Autodesk Inventor part; units mm, degrees
(part 2 of 3)
  spline S242 degree 2 poles (12.9177, 0.2255) (13.1098, 0.3179) (13.6422, 0.3908) (13.9485, 0.4102) knots 0 0 0 1 2 2 2
  line L379 (13.9485, 0.4102) -> (13.9485, 0.4224)
  spline S243 degree 2 poles (13.9485, 0.4224) (13.9485, 0.6096) (13.6714, 0.753) (13.3942, 0.753) knots 0 0 0 1 2 2 2
  spline S244 degree 2 poles (13.3942, 0.753) (13.2702, 0.753) (12.9347, 0.6631) (12.7767, 0.5926) knots 0 0 0 1 2 2 2
  line L380 (12.7767, 0.5926) -> (12.7159, 0.5926)
  line L381 (12.7159, 0.5926) -> (12.7159, 1.1396)
  spline S245 degree 2 poles (12.7159, 1.1396) (12.8205, 1.1688) (13.2872, 1.2514) (13.5255, 1.2514) knots 0 0 0 1 2 2 2
  spline S246 degree 2 poles (13.5255, 1.2514) (14.109, 1.2514) (14.6438, 0.8624) (14.6438, 0.4637) knots 0 0 0 1 2 2 2
  line L382 (14.6438, 0.4637) -> (14.6438, -1.0752)
  line L383 (14.6438, -1.0752) -> (13.9436, -1.0752)
  line L384 (13.9436, -1.0752) -> (13.9436, -0.8345)
  line L385 (13.9436, -0.4844) -> (13.9436, -0.0152)
  spline S247 degree 2 poles (13.9436, -0.0152) (13.7637, -0.0322) (13.5425, -0.059) (13.4355, -0.0979) knots 0 0 0 1 2 2 2
  spline S248 degree 2 poles (13.4355, -0.0979) (13.3407, -0.1295) (13.2386, -0.2607) (13.2386, -0.3677) knots 0 0 0 1 2 2 2
  spline S249 degree 2 poles (13.2386, -0.3677) (13.2386, -0.5257) (13.4112, -0.6449) (13.579, -0.6449) knots 0 0 0 1 2 2 2
  spline S250 degree 2 poles (13.579, -0.6449) (13.6714, -0.6449) (13.8658, -0.5598) (13.9436, -0.4844) knots 0 0 0 1 2 2 2
  line L386 (17.4323, -1.0752) -> (16.5936, -1.0752)
  line L387 (16.5936, -1.0752) -> (15.9809, -0.093)
  line L388 (15.9809, -0.093) -> (15.8715, -0.2389)
  line L389 (15.8715, -0.2389) -> (15.8715, -1.0752)
  line L390 (15.8715, -1.0752) -> (15.1665, -1.0752)
  line L391 (15.1665, -1.0752) -> (15.1665, 2.0585)
  line L392 (15.1665, 2.0585) -> (15.8715, 2.0585)
  line L393 (15.8715, 2.0585) -> (15.8715, 0.3033)
  line L394 (15.8715, 0.3033) -> (16.5401, 1.1882)
  line L395 (16.5401, 1.1882) -> (17.3739, 1.1882)
  line L396 (17.3739, 1.1882) -> (16.5814, 0.2133)
  line L397 (16.5814, 0.2133) -> (17.4323, -1.0752)
  spline S251 degree 2 poles (-23.8578, -3.9603) (-23.8578, -4.1694) (-23.9915, -4.5486) (-24.1155, -4.675) knots 0 0 0 1 2 2 2
  spline S252 degree 2 poles (-24.1155, -4.675) (-24.1909, -4.7553) (-24.3757, -4.8865) (-24.4851, -4.9327) knots 0 0 0 1 2 2 2
  spline S253 degree 2 poles (-24.4851, -4.9327) (-24.5969, -4.9789) (-24.857, -5.0324) (-25.0175, -5.0324) knots 0 0 0 1 2 2 2
  line L398 (-25.0175, -5.0324) -> (-25.4113, -5.0324)
  line L399 (-25.4113, -5.0324) -> (-25.4113, -6.0146)
  line L400 (-25.4113, -6.0146) -> (-26.165, -6.0146)
  line L401 (-26.165, -6.0146) -> (-26.165, -3.0146)
  line L402 (-26.165, -3.0146) -> (-25.0004, -3.0146)
  spline S254 degree 2 poles (-25.0004, -3.0146) (-24.7427, -3.0146) (-24.3659, -3.1094) (-24.2128, -3.2115) knots 0 0 0 1 2 2 2
  spline S255 degree 2 poles (-24.2128, -3.2115) (-24.0426, -3.3258) (-23.8578, -3.7002) (-23.8578, -3.9603) knots 0 0 0 1 2 2 2
  spline S256 degree 2 poles (-24.6309, -3.9797) (-24.6309, -3.8509) (-24.7525, -3.6686) (-24.8351, -3.6345) knots 0 0 0 1 2 2 2
  spline S257 degree 2 poles (-24.8351, -3.6345) (-24.9421, -3.5883) (-25.1366, -3.5737) (-25.3043, -3.5737) knots 0 0 0 1 2 2 2
  line L403 (-25.3043, -3.5737) -> (-25.4113, -3.5737)
  line L404 (-25.4113, -3.5737) -> (-25.4113, -4.4733)
  line L405 (-25.4113, -4.4733) -> (-25.3578, -4.4733)
  spline S258 degree 2 poles (-25.3578, -4.4733) (-25.2533, -4.4733) (-25.0637, -4.4684) (-24.9932, -4.4562) knots 0 0 0 1 2 2 2
  spline S259 degree 2 poles (-24.9932, -4.4562) (-24.9324, -4.4465) (-24.7987, -4.3882) (-24.7622, -4.3517) knots 0 0 0 1 2 2 2
  spline S260 degree 2 poles (-24.7622, -4.3517) (-24.6844, -4.2788) (-24.6309, -4.1159) (-24.6309, -3.9797) knots 0 0 0 1 2 2 2
  spline S261 degree 2 poles (-21.3246, -4.8841) (-21.3246, -5.4433) (-21.9348, -6.0851) (-22.4915, -6.0851) knots 0 0 0 1 2 2 2
  spline S262 degree 2 poles (-22.4915, -6.0851) (-23.0458, -6.0851) (-23.6609, -5.4433) (-23.6609, -4.8841) knots 0 0 0 1 2 2 2
  spline S263 degree 2 poles (-23.6609, -4.8841) (-23.6609, -4.3201) (-23.0458, -3.6807) (-22.4915, -3.6807) knots 0 0 0 1 2 2 2
  spline S264 degree 2 poles (-22.4915, -3.6807) (-21.9372, -3.6807) (-21.3246, -4.3225) (-21.3246, -4.8841) knots 0 0 0 1 2 2 2
  spline S265 degree 2 poles (-22.0466, -4.889) (-22.0466, -4.6872) (-22.1123, -4.4173) (-22.1706, -4.3371) knots 0 0 0 1 2 2 2
  spline S266 degree 2 poles (-22.1706, -4.3371) (-22.2338, -4.252) (-22.3919, -4.1864) (-22.4915, -4.1864) knots 0 0 0 1 2 2 2
  spline S267 degree 2 poles (-22.4915, -4.1864) (-22.5888, -4.1864) (-22.7419, -4.2447) (-22.8051, -4.3274) knots 0 0 0 1 2 2 2
  spline S268 degree 2 poles (-22.8051, -4.3274) (-22.8659, -4.4052) (-22.9389, -4.6799) (-22.9389, -4.889) knots 0 0 0 1 2 2 2
  spline S269 degree 2 poles (-22.9389, -4.889) (-22.9389, -5.0956) (-22.8708, -5.3509) (-22.8149, -5.4287) knots 0 0 0 1 2 2 2
  spline S270 degree 2 poles (-22.8149, -5.4287) (-22.759, -5.5065) (-22.5888, -5.5794) (-22.4867, -5.5794) knots 0 0 0 1 2 2 2
  spline S271 degree 2 poles (-22.4867, -5.5794) (-22.4016, -5.5794) (-22.2265, -5.5065) (-22.1731, -5.4335) knots 0 0 0 1 2 2 2
  spline S272 degree 2 poles (-22.1731, -5.4335) (-22.1123, -5.3485) (-22.0466, -5.1029) (-22.0466, -4.889) knots 0 0 0 1 2 2 2
  line L406 (-18.8935, -6.0146) -> (-19.5985, -6.0146)
  line L407 (-19.5985, -6.0146) -> (-19.5985, -5.7788)
  spline S273 degree 2 poles (-19.5985, -5.7788) (-19.6666, -5.8347) (-19.8416, -5.9635) (-19.9097, -5.9976) knots 0 0 0 1 2 2 2
  spline S274 degree 2 poles (-19.9097, -5.9976) (-19.9923, -6.0365) (-20.1577, -6.0778) (-20.2719, -6.0778) knots 0 0 0 1 2 2 2
  spline S275 degree 2 poles (-20.2719, -6.0778) (-20.6585, -6.0778) (-21.1107, -5.436) (-21.1107, -4.9011) knots 0 0 0 1 2 2 2
  spline S276 degree 2 poles (-21.1107, -4.9011) (-21.1107, -4.6045) (-20.9575, -4.1694) (-20.8238, -4.0089) knots 0 0 0 1 2 2 2
  spline S277 degree 2 poles (-20.8238, -4.0089) (-20.6998, -3.8606) (-20.3497, -3.6904) (-20.1552, -3.6904) knots 0 0 0 1 2 2 2
  spline S278 degree 2 poles (-20.1552, -3.6904) (-19.9778, -3.6904) (-19.7492, -3.7658) (-19.5985, -3.8436) knots 0 0 0 1 2 2 2
  line L408 (-19.5985, -3.8436) -> (-19.5985, -2.8809)
  line L409 (-19.5985, -2.8809) -> (-18.8935, -2.8809)
  line L410 (-18.8935, -2.8809) -> (-18.8935, -6.0146)
  line L411 (-19.5985, -5.3922) -> (-19.5985, -4.2812)
  spline S279 degree 2 poles (-19.5985, -4.2812) (-19.6496, -4.2545) (-19.8197, -4.2204) (-19.8805, -4.2204) knots 0 0 0 1 2 2 2
  spline S280 degree 2 poles (-19.8805, -4.2204) (-20.1333, -4.2204) (-20.3886, -4.5754) (-20.3886, -4.8938) knots 0 0 0 1 2 2 2
  spline S281 degree 2 poles (-20.3886, -4.8938) (-20.3886, -5.2293) (-20.1844, -5.5284) (-19.9583, -5.5284) knots 0 0 0 1 2 2 2
  spline S282 degree 2 poles (-19.9583, -5.5284) (-19.8659, -5.5284) (-19.6763, -5.4554) (-19.5985, -5.3922) knots 0 0 0 1 2 2 2
  spline S283 degree 2 poles (-14.9745, -4.8841) (-14.9745, -5.4433) (-15.5847, -6.0851) (-16.1415, -6.0851) knots 0 0 0 1 2 2 2
  spline S284 degree 2 poles (-16.1415, -6.0851) (-16.6957, -6.0851) (-17.3108, -5.4433) (-17.3108, -4.8841) knots 0 0 0 1 2 2 2
  spline S285 degree 2 poles (-17.3108, -4.8841) (-17.3108, -4.3201) (-16.6957, -3.6807) (-16.1415, -3.6807) knots 0 0 0 1 2 2 2
  spline S286 degree 2 poles (-16.1415, -3.6807) (-15.5872, -3.6807) (-14.9745, -4.3225) (-14.9745, -4.8841) knots 0 0 0 1 2 2 2
  spline S287 degree 2 poles (-15.6966, -4.889) (-15.6966, -4.6872) (-15.7622, -4.4173) (-15.8205, -4.3371) knots 0 0 0 1 2 2 2
  spline S288 degree 2 poles (-15.8205, -4.3371) (-15.8838, -4.252) (-16.0418, -4.1864) (-16.1415, -4.1864) knots 0 0 0 1 2 2 2
  spline S289 degree 2 poles (-16.1415, -4.1864) (-16.2387, -4.1864) (-16.3919, -4.2447) (-16.4551, -4.3274) knots 0 0 0 1 2 2 2
  spline S290 degree 2 poles (-16.4551, -4.3274) (-16.5158, -4.4052) (-16.5888, -4.6799) (-16.5888, -4.889) knots 0 0 0 1 2 2 2
  spline S291 degree 2 poles (-16.5888, -4.889) (-16.5888, -5.0956) (-16.5207, -5.3509) (-16.4648, -5.4287) knots 0 0 0 1 2 2 2
  spline S292 degree 2 poles (-16.4648, -5.4287) (-16.4089, -5.5065) (-16.2387, -5.5794) (-16.1366, -5.5794) knots 0 0 0 1 2 2 2
  spline S293 degree 2 poles (-16.1366, -5.5794) (-16.0515, -5.5794) (-15.8765, -5.5065) (-15.823, -5.4335) knots 0 0 0 1 2 2 2
  spline S294 degree 2 poles (-15.823, -5.4335) (-15.7622, -5.3485) (-15.6966, -5.1029) (-15.6966, -4.889) knots 0 0 0 1 2 2 2
  spline S295 degree 2 poles (-12.3829, -4.8525) (-12.3829, -5.3947) (-12.9324, -6.0583) (-13.3359, -6.0583) knots 0 0 0 1 2 2 2
  spline S296 degree 2 poles (-13.3359, -6.0583) (-13.5037, -6.0583) (-13.7541, -5.983) (-13.8951, -5.9003) knots 0 0 0 1 2 2 2
  line L412 (-13.8951, -5.9003) -> (-13.8951, -6.8436)
  line L413 (-13.8951, -6.8436) -> (-14.6001, -6.8436)
  line L414 (-14.6001, -6.8436) -> (-14.6001, -3.7512)
  line L415 (-14.6001, -3.7512) -> (-13.8951, -3.7512)
  line L416 (-13.8951, -3.7512) -> (-13.8951, -3.9895)
  spline S297 degree 2 poles (-13.8951, -3.9895) (-13.7395, -3.8558) (-13.4186, -3.6904) (-13.2071, -3.6904) knots 0 0 0 1 2 2 2
  spline S298 degree 2 poles (-13.2071, -3.6904) (-12.8133, -3.6904) (-12.3829, -4.3152) (-12.3829, -4.8525) knots 0 0 0 1 2 2 2
  spline S299 degree 2 poles (-13.105, -4.8671) (-13.105, -4.5365) (-13.3092, -4.2399) (-13.5231, -4.2399) knots 0 0 0 1 2 2 2
  spline S300 degree 2 poles (-13.5231, -4.2399) (-13.618, -4.2399) (-13.8051, -4.3006) (-13.8951, -4.3614) knots 0 0 0 1 2 2 2
  line L417 (-13.8951, -4.3614) -> (-13.8951, -5.4968)
  spline S301 degree 2 poles (-13.8951, -5.4968) (-13.8392, -5.5211) (-13.703, -5.5405) (-13.6107, -5.5405) knots 0 0 0 1 2 2 2
  spline S302 degree 2 poles (-13.6107, -5.5405) (-13.3554, -5.5405) (-13.105, -5.205) (-13.105, -4.8671) knots 0 0 0 1 2 2 2
  line L418 (-11.2987, -6.0146) -> (-12.0037, -6.0146)
  line L419 (-12.0037, -6.0146) -> (-12.0037, -3.7512)
  line L420 (-12.0037, -3.7512) -> (-11.2987, -3.7512)
  line L421 (-11.2987, -3.7512) -> (-11.2987, -6.0146)
  line L422 (-11.2768, -3.4279) -> (-12.0231, -3.4279)
  line L423 (-12.0231, -3.4279) -> (-12.0231, -2.8784)
  line L424 (-12.0231, -2.8784) -> (-11.2768, -2.8784)
  line L425 (-11.2768, -2.8784) -> (-11.2768, -3.4279)
  spline S303 degree 2 poles (-9.5993, -6.0754) (-10.2411, -6.0754) (-10.9243, -5.4627) (-10.9243, -4.8963) knots 0 0 0 1 2 2 2
  spline S304 degree 2 poles (-10.9243, -4.8963) (-10.9243, -4.342) (-10.2873, -3.6807) (-9.7136, -3.6807) knots 0 0 0 1 2 2 2
  spline S305 degree 2 poles (-9.7136, -3.6807) (-9.1957, -3.6807) (-8.6706, -4.2423) (-8.6706, -4.7626) knots 0 0 0 1 2 2 2
  line L426 (-8.6706, -4.7626) -> (-8.6706, -5.0178)
  line L427 (-8.6706, -5.0178) -> (-10.2192, -5.0178)
  spline S306 degree 2 poles (-10.2192, -5.0178) (-10.2095, -5.1758) (-10.0953, -5.3849) (-10.0029, -5.4481) knots 0 0 0 1 2 2 2
  spline S307 degree 2 poles (-10.0029, -5.4481) (-9.9129, -5.5113) (-9.6698, -5.5648) (-9.5264, -5.5648) knots 0 0 0 1 2 2 2
  spline S308 degree 2 poles (-9.5264, -5.5648) (-9.4048, -5.5648) (-9.1666, -5.5113) (-9.0669, -5.4652) knots 0 0 0 1 2 2 2
  spline S309 degree 2 poles (-9.0669, -5.4652) (-8.9794, -5.4287) (-8.8335, -5.3387) (-8.7873, -5.3047) knots 0 0 0 1 2 2 2
  line L428 (-8.7873, -5.3047) -> (-8.712, -5.3047)
  line L429 (-8.712, -5.3047) -> (-8.712, -5.8882)
  spline S310 degree 2 poles (-8.712, -5.8882) (-8.7995, -5.9222) (-8.9405, -5.9805) (-9.0669, -6.0097) knots 0 0 0 1 2 2 2
  spline S311 degree 2 poles (-9.0669, -6.0097) (-9.1812, -6.0413) (-9.4243, -6.0754) (-9.5993, -6.0754) knots 0 0 0 1 2 2 2
  spline S312 degree 2 poles (-9.3659, -4.5924) (-9.3708, -4.3687) (-9.5677, -4.1329) (-9.7695, -4.1329) knots 0 0 0 1 2 2 2
  spline S313 degree 2 poles (-9.7695, -4.1329) (-9.9761, -4.1329) (-10.2095, -4.3809) (-10.2217, -4.5924) knots 0 0 0 1 2 2 2
  line L430 (-10.2217, -4.5924) -> (-9.3659, -4.5924)
  line L431 (-6.0426, -6.0146) -> (-6.8813, -6.0146)
  line L432 (-6.8813, -6.0146) -> (-7.494, -5.0324)
  line L433 (-7.494, -5.0324) -> (-7.6034, -5.1783)
  line L434 (-7.6034, -5.1783) -> (-7.6034, -6.0146)
  line L435 (-7.6034, -6.0146) -> (-8.3084, -6.0146)
  line L436 (-8.3084, -6.0146) -> (-8.3084, -2.8809)
  line L437 (-8.3084, -2.8809) -> (-7.6034, -2.8809)
  line L438 (-7.6034, -2.8809) -> (-7.6034, -4.6361)
  line L439 (-7.6034, -4.6361) -> (-6.9348, -3.7512)
  line L440 (-6.9348, -3.7512) -> (-6.1009, -3.7512)
  line L441 (-6.1009, -3.7512) -> (-6.8935, -4.7261)
  line L442 (-6.8935, -4.7261) -> (-6.0426, -6.0146)
  spline S314 degree 2 poles (-4.5742, -5.7739) (-4.6471, -5.8347) (-4.7614, -5.9319) (-4.8586, -5.9805) knots 0 0 0 1 2 2 2
  spline S315 degree 2 poles (-4.8586, -5.9805) (-4.9534, -6.0267) (-5.1333, -6.0754) (-5.2938, -6.0754) knots 0 0 0 1 2 2 2
  spline S316 degree 2 poles (-5.2938, -6.0754) (-5.5953, -6.0754) (-5.9915, -5.6718) (-5.9915, -5.3655) knots 0 0 0 1 2 2 2
  spline S317 degree 2 poles (-5.9915, -5.3655) (-5.9915, -5.1151) (-5.7898, -4.8039) (-5.6001, -4.7139) knots 0 0 0 1 2 2 2
  spline S318 degree 2 poles (-5.6001, -4.7139) (-5.4081, -4.6216) (-4.8757, -4.5486) (-4.5693, -4.5292) knots 0 0 0 1 2 2 2
  line L443 (-4.5693, -4.5292) -> (-4.5693, -4.517)
  spline S319 degree 2 poles (-4.5693, -4.517) (-4.5693, -4.3298) (-4.8465, -4.1864) (-5.1236, -4.1864) knots 0 0 0 1 2 2 2
  spline S320 degree 2 poles (-5.1236, -4.1864) (-5.2476, -4.1864) (-5.5831, -4.2763) (-5.7411, -4.3468) knots 0 0 0 1 2 2 2
  line L444 (-5.7411, -4.3468) -> (-5.8019, -4.3468)
  line L445 (-5.8019, -4.3468) -> (-5.8019, -3.7998)
  spline S321 degree 2 poles (-5.8019, -3.7998) (-5.6974, -3.7707) (-5.2306, -3.688) (-4.9923, -3.688) knots 0 0 0 1 2 2 2
  spline S322 degree 2 poles (-4.9923, -3.688) (-4.4089, -3.688) (-3.874, -4.077) (-3.874, -4.4757) knots 0 0 0 1 2 2 2
  line L446 (-3.874, -4.4757) -> (-3.874, -6.0146)
  line L447 (-3.874, -6.0146) -> (-4.5742, -6.0146)
  line L448 (-4.5742, -6.0146) -> (-4.5742, -5.7739)
  spline S323 degree 2 poles (-4.0102, -6.0146) (-4.0855, -6.0729) (-4.1585, -6.1994) (-4.1585, -6.2577) knots 0 0 0 1 2 2 2
  spline S324 degree 2 poles (-4.1585, -6.2577) (-4.1585, -6.282) (-4.1439, -6.3258) (-4.1269, -6.3452) knots 0 0 0 1 2 2 2
  spline S325 degree 2 poles (-4.1269, -6.3452) (-4.105, -6.3671) (-4.0588, -6.389) (-4.015, -6.389) knots 0 0 0 1 2 2 2
  spline S326 degree 2 poles (-4.015, -6.389) (-3.9859, -6.389) (-3.9154, -6.372) (-3.891, -6.3647) knots 0 0 0 1 2 2 2
  line L449 (-3.891, -6.3647) -> (-3.8716, -6.3647)
  line L450 (-3.8716, -6.3647) -> (-3.8716, -6.7828)
  spline S327 degree 2 poles (-3.8716, -6.7828) (-3.9543, -6.8144) (-4.1706, -6.8436) (-4.2338, -6.8436) knots 0 0 0 1 2 2 2
  spline S328 degree 2 poles (-4.2338, -6.8436) (-4.4235, -6.8436) (-4.6593, -6.6442) (-4.6593, -6.4959) knots 0 0 0 1 2 2 2
  spline S329 degree 2 poles (-4.6593, -6.4959) (-4.6593, -6.3428) (-4.5134, -6.0899) (-4.4259, -6.0146) knots 0 0 0 1 2 2 2
  line L451 (-4.4259, -6.0146) -> (-4.0102, -6.0146)
  line L452 (-4.5742, -5.4238) -> (-4.5742, -4.9546)
  spline S330 degree 2 poles (-4.5742, -4.9546) (-4.7541, -4.9716) (-4.9753, -4.9984) (-5.0823, -5.0373) knots 0 0 0 1 2 2 2
  spline S331 degree 2 poles (-5.0823, -5.0373) (-5.1771, -5.0689) (-5.2792, -5.2002) (-5.2792, -5.3071) knots 0 0 0 1 2 2 2
  spline S332 degree 2 poles (-5.2792, -5.3071) (-5.2792, -5.4652) (-5.1066, -5.5843) (-4.9389, -5.5843) knots 0 0 0 1 2 2 2
  spline S333 degree 2 poles (-4.9389, -5.5843) (-4.8465, -5.5843) (-4.652, -5.4992) (-4.5742, -5.4238) knots 0 0 0 1 2 2 2
  line L453 (0.5579, -6.0146) -> (0.5579, -4.8841)
  spline S334 degree 2 poles (0.5579, -4.8841) (0.5579, -4.7164) (0.5457, -4.4878) (0.5166, -4.4149) knots 0 0 0 1 2 2 2
  spline S335 degree 2 poles (0.5166, -4.4149) (0.485, -4.342) (0.3585, -4.2763) (0.2443, -4.2763) knots 0 0 0 1 2 2 2
  spline S336 degree 2 poles (0.2443, -4.2763) (0.1641, -4.2763) (0.0085, -4.3468) (-0.0839, -4.4125) knots 0 0 0 1 2 2 2
  line L454 (-0.0839, -4.4125) -> (-0.0839, -6.0146)
  line L455 (-0.0839, -6.0146) -> (-0.7938, -6.0146)
  line L456 (-0.7938, -6.0146) -> (-0.7938, -4.8841)
  spline S337 degree 2 poles (-0.7938, -4.8841) (-0.7938, -4.7188) (-0.8084, -4.4878) (-0.8376, -4.4149) knots 0 0 0 1 2 2 2
  spline S338 degree 2 poles (-0.8376, -4.4149) (-0.8692, -4.342) (-0.9956, -4.2763) (-1.1098, -4.2763) knots 0 0 0 1 2 2 2
  spline S339 degree 2 poles (-1.1098, -4.2763) (-1.1949, -4.2763) (-1.3627, -4.3566) (-1.4405, -4.4125) knots 0 0 0 1 2 2 2
  line L457 (-1.4405, -4.4125) -> (-1.4405, -6.0146)
  line L458 (-1.4405, -6.0146) -> (-2.1455, -6.0146)
  line L459 (-2.1455, -6.0146) -> (-2.1455, -3.7512)
  line L460 (-2.1455, -3.7512) -> (-1.4405, -3.7512)
  line L461 (-1.4405, -3.7512) -> (-1.4405, -4.0016)
  spline S340 degree 2 poles (-1.4405, -4.0016) (-1.2679, -3.8558) (-0.9591, -3.6904) (-0.7671, -3.6904) knots 0 0 0 1 2 2 2
  spline S341 degree 2 poles (-0.7671, -3.6904) (-0.5604, -3.6904) (-0.2444, -3.8874) (-0.1617, -4.0843) knots 0 0 0 1 2 2 2
  spline S342 degree 2 poles (-0.1617, -4.0843) (0.0401, -3.8947) (0.3999, -3.6904) (0.5846, -3.6904) knots 0 0 0 1 2 2 2
  spline S343 degree 2 poles (0.5846, -3.6904) (0.7427, -3.6904) (0.9931, -3.7901) (1.0782, -3.8922) knots 0 0 0 1 2 2 2
  spline S344 degree 2 poles (1.0782, -3.8922) (1.173, -4.0016) (1.2678, -4.3006) (1.2678, -4.5413) knots 0 0 0 1 2 2 2
  line L462 (1.2678, -4.5413) -> (1.2678, -6.0146)
  line L463 (1.2678, -6.0146) -> (0.5579, -6.0146)
  spline S345 degree 2 poles (2.9501, -6.0754) (2.3083, -6.0754) (1.6252, -5.4627) (1.6252, -4.8963) knots 0 0 0 1 2 2 2
  spline S346 degree 2 poles (1.6252, -4.8963) (1.6252, -4.342) (2.2621, -3.6807) (2.8359, -3.6807) knots 0 0 0 1 2 2 2
  spline S347 degree 2 poles (2.8359, -3.6807) (3.3537, -3.6807) (3.8788, -4.2423) (3.8788, -4.7626) knots 0 0 0 1 2 2 2
  line L464 (3.8788, -4.7626) -> (3.8788, -5.0178)
  line L465 (3.8788, -5.0178) -> (2.3302, -5.0178)
  spline S348 degree 2 poles (2.3302, -5.0178) (2.3399, -5.1758) (2.4542, -5.3849) (2.5466, -5.4481) knots 0 0 0 1 2 2 2
  spline S349 degree 2 poles (2.5466, -5.4481) (2.6365, -5.5113) (2.8796, -5.5648) (3.0231, -5.5648) knots 0 0 0 1 2 2 2
  spline S350 degree 2 poles (3.0231, -5.5648) (3.1446, -5.5648) (3.3829, -5.5113) (3.4825, -5.4652) knots 0 0 0 1 2 2 2
  spline S351 degree 2 poles (3.4825, -5.4652) (3.5701, -5.4287) (3.7159, -5.3387) (3.7621, -5.3047) knots 0 0 0 1 2 2 2
  line L466 (3.7621, -5.3047) -> (3.8375, -5.3047)
  line L467 (3.8375, -5.3047) -> (3.8375, -5.8882)
  spline S352 degree 2 poles (3.8375, -5.8882) (3.75, -5.9222) (3.609, -5.9805) (3.4825, -6.0097) knots 0 0 0 1 2 2 2
  spline S353 degree 2 poles (3.4825, -6.0097) (3.3683, -6.0413) (3.1252, -6.0754) (2.9501, -6.0754) knots 0 0 0 1 2 2 2
  spline S354 degree 2 poles (3.1835, -4.5924) (3.1786, -4.3687) (2.9817, -4.1329) (2.7799, -4.1329) knots 0 0 0 1 2 2 2
  spline S355 degree 2 poles (2.7799, -4.1329) (2.5733, -4.1329) (2.3399, -4.3809) (2.3278, -4.5924) knots 0 0 0 1 2 2 2
  line L468 (2.3278, -4.5924) -> (3.1835, -4.5924)
  line L469 (5.7605, -4.4198) -> (5.7021, -4.4198)
  spline S356 degree 2 poles (5.7021, -4.4198) (5.6608, -4.4052) (5.5077, -4.3906) (5.4153, -4.3906) knots 0 0 0 1 2 2 2
  spline S357 degree 2 poles (5.4153, -4.3906) (5.3059, -4.3906) (5.0603, -4.4562) (4.9461, -4.5) knots 0 0 0 1 2 2 2
  line L470 (4.9461, -4.5) -> (4.9461, -6.0146)
  line L471 (4.9461, -6.0146) -> (4.241, -6.0146)
  line L472 (4.241, -6.0146) -> (4.241, -3.7512)
  line L473 (4.241, -3.7512) -> (4.9461, -3.7512)
  line L474 (4.9461, -3.7512) -> (4.9461, -4.077)
  spline S358 degree 2 poles (4.9461, -4.077) (4.9947, -4.0332) (5.1649, -3.8971) (5.2354, -3.8558) knots 0 0 0 1 2 2 2
  spline S359 degree 2 poles (5.2354, -3.8558) (5.3132, -3.8096) (5.5174, -3.7439) (5.6073, -3.7439) knots 0 0 0 1 2 2 2
  spline S360 degree 2 poles (5.6073, -3.7439) (5.6414, -3.7439) (5.7265, -3.7488) (5.7605, -3.7512) knots 0 0 0 1 2 2 2
  line L475 (5.7605, -3.7512) -> (5.7605, -4.4198)
  line L476 (8.1406, -3.7512) -> (7.0004, -6.8436)
  line L477 (7.0004, -6.8436) -> (6.2419, -6.8436)
  line L478 (6.2419, -6.8436) -> (6.5846, -5.9587)
  line L479 (6.5846, -5.9587) -> (5.7556, -3.7512)
  line L480 (5.7556, -3.7512) -> (6.4947, -3.7512)
  line L481 (6.4947, -3.7512) -> (6.9712, -5.171)
  line L482 (6.9712, -5.171) -> (7.4161, -3.7512)
  line L483 (7.4161, -3.7512) -> (8.1406, -3.7512)
  spline S361 degree 2 poles (9.271, -6.0583) (8.8407, -6.0583) (8.4469, -5.7034) (8.4469, -5.2998) knots 0 0 0 1 2 2 2
  line L484 (8.4469, -5.2998) -> (8.4469, -4.2423)
  line L485 (8.4469, -4.2423) -> (8.177, -4.2423)
  line L486 (8.177, -4.2423) -> (8.177, -3.7512)
  line L487 (8.177, -3.7512) -> (8.4469, -3.7512)
  line L488 (8.4469, -3.7512) -> (8.4469, -3.1045)
  line L489 (8.4469, -3.1045) -> (9.1519, -3.1045)
  line L490 (9.1519, -3.1045) -> (9.1519, -3.7512)
  line L491 (9.1519, -3.7512) -> (9.8326, -3.7512)
  line L492 (9.8326, -3.7512) -> (9.8326, -4.2423)
  line L493 (9.8326, -4.2423) -> (9.1519, -4.2423)
  line L494 (9.1519, -4.2423) -> (9.1519, -5.047)
  spline S362 degree 2 poles (9.1519, -5.047) (9.1519, -5.1661) (9.1568, -5.3436) (9.1859, -5.4141) knots 0 0 0 1 2 2 2
  spline S363 degree 2 poles (9.1859, -5.4141) (9.2151, -5.4846) (9.3585, -5.5673) (9.4947, -5.5673) knots 0 0 0 1 2 2 2
  spline S364 degree 2 poles (9.4947, -5.5673) (9.553, -5.5673) (9.7354, -5.5186) (9.7718, -5.4992) knots 0 0 0 1 2 2 2
  line L495 (9.7718, -5.4992) -> (9.8326, -5.4992)
  line L496 (9.8326, -5.4992) -> (9.8326, -5.9951)
  spline S365 degree 2 poles (9.8326, -5.9951) (9.7184, -6.0243) (9.4607, -6.0583) (9.271, -6.0583) knots 0 0 0 1 2 2 2
  spline S366 degree 2 poles (12.2905, -4.8841) (12.2905, -5.4433) (11.6803, -6.0851) (11.1235, -6.0851) knots 0 0 0 1 2 2 2
  spline S367 degree 2 poles (11.1235, -6.0851) (10.5692, -6.0851) (9.9542, -5.4433) (9.9542, -4.8841) knots 0 0 0 1 2 2 2
  spline S368 degree 2 poles (9.9542, -4.8841) (9.9542, -4.3201) (10.5692, -3.6807) (11.1235, -3.6807) knots 0 0 0 1 2 2 2
  spline S369 degree 2 poles (11.1235, -3.6807) (11.6778, -3.6807) (12.2905, -4.3225) (12.2905, -4.8841) knots 0 0 0 1 2 2 2
  spline S370 degree 2 poles (11.5684, -4.889) (11.5684, -4.6872) (11.5028, -4.4173) (11.4444, -4.3371) knots 0 0 0 1 2 2 2
  spline S371 degree 2 poles (11.4444, -4.3371) (11.3812, -4.252) (11.2232, -4.1864) (11.1235, -4.1864) knots 0 0 0 1 2 2 2
  spline S372 degree 2 poles (11.1235, -4.1864) (11.0263, -4.1864) (10.8731, -4.2447) (10.8099, -4.3274) knots 0 0 0 1 2 2 2
  spline S373 degree 2 poles (10.8099, -4.3274) (10.7491, -4.4052) (10.6762, -4.6799) (10.6762, -4.889) knots 0 0 0 1 2 2 2
  spline S374 degree 2 poles (10.6762, -4.889) (10.6762, -5.0956) (10.7443, -5.3509) (10.8002, -5.4287) knots 0 0 0 1 2 2 2
  spline S375 degree 2 poles (10.8002, -5.4287) (10.8561, -5.5065) (11.0263, -5.5794) (11.1284, -5.5794) knots 0 0 0 1 2 2 2
  spline S376 degree 2 poles (11.1284, -5.5794) (11.2135, -5.5794) (11.3885, -5.5065) (11.442, -5.4335) knots 0 0 0 1 2 2 2
  spline S377 degree 2 poles (11.442, -5.4335) (11.5028, -5.3485) (11.5684, -5.1029) (11.5684, -4.889) knots 0 0 0 1 2 2 2
  line L497 (14.1843, -4.4198) -> (14.126, -4.4198)
  spline S378 degree 2 poles (14.126, -4.4198) (14.0846, -4.4052) (13.9315, -4.3906) (13.8391, -4.3906) knots 0 0 0 1 2 2 2
  spline S379 degree 2 poles (13.8391, -4.3906) (13.7297, -4.3906) (13.4842, -4.4562) (13.3699, -4.5) knots 0 0 0 1 2 2 2
  line L498 (13.3699, -4.5) -> (13.3699, -6.0146)
  line L499 (13.3699, -6.0146) -> (12.6649, -6.0146)
  line L500 (12.6649, -6.0146) -> (12.6649, -3.7512)
  line L501 (12.6649, -3.7512) -> (13.3699, -3.7512)
  line L502 (13.3699, -3.7512) -> (13.3699, -4.077)
  spline S380 degree 2 poles (13.3699, -4.077) (13.4185, -4.0332) (13.5887, -3.8971) (13.6592, -3.8558) knots 0 0 0 1 2 2 2
  spline S381 degree 2 poles (13.6592, -3.8558) (13.737, -3.8096) (13.9412, -3.7439) (14.0312, -3.7439) knots 0 0 0 1 2 2 2
  spline S382 degree 2 poles (14.0312, -3.7439) (14.0652, -3.7439) (14.1503, -3.7488) (14.1843, -3.7512) knots 0 0 0 1 2 2 2
  line L503 (14.1843, -3.7512) -> (14.1843, -4.4198)
  line L504 (16.5644, -3.7512) -> (15.4242, -6.8436)
  line L505 (15.4242, -6.8436) -> (14.6657, -6.8436)
  line L506 (14.6657, -6.8436) -> (15.0085, -5.9587)
  line L507 (15.0085, -5.9587) -> (14.1795, -3.7512)
  line L508 (14.1795, -3.7512) -> (14.9185, -3.7512)
  line L509 (14.9185, -3.7512) -> (15.395, -5.171)
  line L510 (15.395, -5.171) -> (15.8399, -3.7512)
  line L511 (15.8399, -3.7512) -> (16.5644, -3.7512)
  spline S383 degree 2 poles (17.938, -6.0754) (17.6584, -6.0754) (17.194, -5.9344) (17.0214, -5.7885) knots 0 0 0 1 2 2 2
  spline S384 degree 2 poles (17.0214, -5.7885) (16.8537, -5.6402) (16.6641, -5.1953) (16.6641, -4.8938) knots 0 0 0 1 2 2 2
  spline S385 degree 2 poles (16.6641, -4.8938) (16.6641, -4.5681) (16.8683, -4.1135) (17.0457, -3.9676) knots 0 0 0 1 2 2 2
  spline S386 degree 2 poles (17.0457, -3.9676) (17.2135, -3.8266) (17.6705, -3.6904) (17.9185, -3.6904) knots 0 0 0 1 2 2 2
  spline S387 degree 2 poles (17.9185, -3.6904) (18.1057, -3.6904) (18.4801, -3.778) (18.6697, -3.8728) knots 0 0 0 1 2 2 2
  line L512 (18.6697, -3.8728) -> (18.6697, -4.4757)
  line L513 (18.6697, -4.4757) -> (18.5798, -4.4757)
  spline S388 degree 2 poles (18.5798, -4.4757) (18.536, -4.4344) (18.4145, -4.3371) (18.3415, -4.2982) knots 0 0 0 1 2 2 2
  spline S389 degree 2 poles (18.3415, -4.2982) (18.2637, -4.2545) (18.0717, -4.1961) (17.9526, -4.1961) knots 0 0 0 1 2 2 2
  spline S390 degree 2 poles (17.9526, -4.1961) (17.6827, -4.1961) (17.3861, -4.5729) (17.3861, -4.8938) knots 0 0 0 1 2 2 2
  spline S391 degree 2 poles (17.3861, -4.8938) (17.3861, -5.2342) (17.7021, -5.5697) (17.9647, -5.5697) knots 0 0 0 1 2 2 2
  spline S392 degree 2 poles (17.9647, -5.5697) (18.0984, -5.5697) (18.2978, -5.5089) (18.3707, -5.4652) knots 0 0 0 1 2 2 2
  spline S393 degree 2 poles (18.3707, -5.4652) (18.4412, -5.4238) (18.5433, -5.3314) (18.5798, -5.295) knots 0 0 0 1 2 2 2
  line L514 (18.5798, -5.295) -> (18.6697, -5.295)
  line L515 (18.6697, -5.295) -> (18.6697, -5.9003)
  spline S394 degree 2 poles (18.6697, -5.9003) (18.609, -5.9271) (18.4509, -5.9951) (18.3683, -6.017) knots 0 0 0 1 2 2 2
  spline S395 degree 2 poles (18.3683, -6.017) (18.2662, -6.0462) (18.0863, -6.0754) (17.938, -6.0754) knots 0 0 0 1 2 2 2
  line L516 (20.8091, -6.0146) -> (18.8326, -6.0146)
  line L517 (18.8326, -6.0146) -> (18.8326, -5.5502)
  line L518 (18.8326, -5.5502) -> (19.912, -4.2812)
  line L519 (19.912, -4.2812) -> (18.8812, -4.2812)
  line L520 (18.8812, -4.2812) -> (18.8812, -3.7512)
  line L521 (18.8812, -3.7512) -> (20.7872, -3.7512)
  line L522 (20.7872, -3.7512) -> (20.7872, -4.2083)
  line L523 (20.7872, -4.2083) -> (19.7054, -5.4749)
  line L524 (19.7054, -5.4749) -> (20.8091, -5.4749)
  line L525 (20.8091, -5.4749) -> (20.8091, -6.0146)
  line L526 (23.2913, -6.0146) -> (22.5814, -6.0146)
  line L527 (22.5814, -6.0146) -> (22.5814, -4.8938)
  spline S396 degree 2 poles (22.5814, -4.8938) (22.5814, -4.7553) (22.5595, -4.483) (22.5303, -4.4198) knots 0 0 0 1 2 2 2
  spline S397 degree 2 poles (22.5303, -4.4198) (22.4939, -4.342) (22.3577, -4.2763) (22.241, -4.2763) knots 0 0 0 1 2 2 2
  spline S398 degree 2 poles (22.241, -4.2763) (22.156, -4.2763) (21.9785, -4.342) (21.8788, -4.4125) knots 0 0 0 1 2 2 2
  line L528 (21.8788, -4.4125) -> (21.8788, -6.0146)
  line L529 (21.8788, -6.0146) -> (21.1738, -6.0146)
  line L530 (21.1738, -6.0146) -> (21.1738, -3.7512)
  line L531 (21.1738, -3.7512) -> (21.8788, -3.7512)
  line L532 (21.8788, -3.7512) -> (21.8788, -4.0016)
  spline S399 degree 2 poles (21.8788, -4.0016) (22.0514, -3.8558) (22.3796, -3.6904) (22.579, -3.6904) knots 0 0 0 1 2 2 2
  spline S400 degree 2 poles (22.579, -3.6904) (22.9242, -3.6904) (23.2913, -4.128) (23.2913, -4.5413) knots 0 0 0 1 2 2 2
  line L533 (23.2913, -4.5413) -> (23.2913, -6.0146)
  spline S401 degree 2 poles (25.0611, -5.7739) (24.9882, -5.8347) (24.8739, -5.9319) (24.7767, -5.9805) knots 0 0 0 1 2 2 2
  spline S402 degree 2 poles (24.7767, -5.9805) (24.6819, -6.0267) (24.502, -6.0754) (24.3415, -6.0754) knots 0 0 0 1 2 2 2
  spline S403 degree 2 poles (24.3415, -6.0754) (24.0401, -6.0754) (23.6438, -5.6718) (23.6438, -5.3655) knots 0 0 0 1 2 2 2
  spline S404 degree 2 poles (23.6438, -5.3655) (23.6438, -5.1151) (23.8456, -4.8039) (24.0352, -4.7139) knots 0 0 0 1 2 2 2
  spline S405 degree 2 poles (24.0352, -4.7139) (24.2273, -4.6216) (24.7597, -4.5486) (25.066, -4.5292) knots 0 0 0 1 2 2 2
  line L534 (25.066, -4.5292) -> (25.066, -4.517)
  spline S406 degree 2 poles (25.066, -4.517) (25.066, -4.3298) (24.7889, -4.1864) (24.5117, -4.1864) knots 0 0 0 1 2 2 2
  spline S407 degree 2 poles (24.5117, -4.1864) (24.3877, -4.1864) (24.0522, -4.2763) (23.8942, -4.3468) knots 0 0 0 1 2 2 2
  line L535 (23.8942, -4.3468) -> (23.8334, -4.3468)
  line L536 (23.8334, -4.3468) -> (23.8334, -3.7998)
  spline S408 degree 2 poles (23.8334, -3.7998) (23.938, -3.7707) (24.4047, -3.688) (24.643, -3.688) knots 0 0 0 1 2 2 2
  spline S409 degree 2 poles (24.643, -3.688) (25.2265, -3.688) (25.7613, -4.077) (25.7613, -4.4757) knots 0 0 0 1 2 2 2
  line L537 (25.7613, -4.4757) -> (25.7613, -6.0146)
  line L538 (25.7613, -6.0146) -> (25.0611, -6.0146)
  line L539 (25.0611, -6.0146) -> (25.0611, -5.7739)
  spline S410 degree 2 poles (25.6252, -6.0146) (25.5498, -6.0729) (25.4769, -6.1994) (25.4769, -6.2577) knots 0 0 0 1 2 2 2
  spline S411 degree 2 poles (25.4769, -6.2577) (25.4769, -6.282) (25.4914, -6.3258) (25.5085, -6.3452) knots 0 0 0 1 2 2 2
  spline S412 degree 2 poles (25.5085, -6.3452) (25.5303, -6.3671) (25.5765, -6.389) (25.6203, -6.389) knots 0 0 0 1 2 2 2
  spline S413 degree 2 poles (25.6203, -6.389) (25.6495, -6.389) (25.72, -6.372) (25.7443, -6.3647) knots 0 0 0 1 2 2 2
  line L540 (25.7443, -6.3647) -> (25.7637, -6.3647)
  line L541 (25.7637, -6.3647) -> (25.7637, -6.7828)
  spline S414 degree 2 poles (25.7637, -6.7828) (25.6811, -6.8144) (25.4647, -6.8436) (25.4015, -6.8436) knots 0 0 0 1 2 2 2
  spline S415 degree 2 poles (25.4015, -6.8436) (25.2119, -6.8436) (24.9761, -6.6442) (24.9761, -6.4959) knots 0 0 0 1 2 2 2
  spline S416 degree 2 poles (24.9761, -6.4959) (24.9761, -6.3428) (25.1219, -6.0899) (25.2094, -6.0146) knots 0 0 0 1 2 2 2
  line L542 (25.2094, -6.0146) -> (25.6252, -6.0146)
  line L543 (25.0611, -5.4238) -> (25.0611, -4.9546)
  spline S417 degree 2 poles (25.0611, -4.9546) (24.8812, -4.9716) (24.66, -4.9984) (24.553, -5.0373) knots 0 0 0 1 2 2 2
  spline S418 degree 2 poles (24.553, -5.0373) (24.4582, -5.0689) (24.3561, -5.2002) (24.3561, -5.3071) knots 0 0 0 1 2 2 2
  spline S419 degree 2 poles (24.3561, -5.3071) (24.3561, -5.4652) (24.5287, -5.5843) (24.6965, -5.5843) knots 0 0 0 1 2 2 2
  spline S420 degree 2 poles (24.6965, -5.5843) (24.7889, -5.5843) (24.9833, -5.4992) (25.0611, -5.4238) knots 0 0 0 1 2 2 2
  line L544 (27.1203, -6.0146) -> (26.408, -6.0146)
  line L545 (26.408, -6.0146) -> (26.408, -5.222)
  line L546 (26.408, -5.222) -> (27.1203, -5.222)
  line L547 (27.1203, -5.222) -> (27.1203, -6.0146)
  line L548 (27.1203, -4.5438) -> (26.408, -4.5438)
  line L549 (26.408, -4.5438) -> (26.408, -3.7512)
  line L550 (26.408, -3.7512) -> (27.1203, -3.7512)
  line L551 (27.1203, -3.7512) -> (27.1203, -4.5438)
  line L552 (-28.7116, -10.954) -> (-29.4166, -10.954)
  line L553 (-29.4166, -10.954) -> (-29.4166, -10.7182)
  spline S421 degree 2 poles (-29.4166, -10.7182) (-29.4846, -10.7741) (-29.6597, -10.903) (-29.7278, -10.937) knots 0 0 0 1 2 2 2
  spline S422 degree 2 poles (-29.7278, -10.937) (-29.8104, -10.9759) (-29.9757, -11.0172) (-30.09, -11.0172) knots 0 0 0 1 2 2 2
  spline S423 degree 2 poles (-30.09, -11.0172) (-30.4765, -11.0172) (-30.9287, -10.3754) (-30.9287, -9.8406) knots 0 0 0 1 2 2 2
  spline S424 degree 2 poles (-30.9287, -9.8406) (-30.9287, -9.544) (-30.7756, -9.1088) (-30.6419, -8.9483) knots 0 0 0 1 2 2 2
  spline S425 degree 2 poles (-30.6419, -8.9483) (-30.5179, -8.8) (-30.1678, -8.6299) (-29.9733, -8.6299) knots 0 0 0 1 2 2 2
  spline S426 degree 2 poles (-29.9733, -8.6299) (-29.7958, -8.6299) (-29.5673, -8.7052) (-29.4166, -8.783) knots 0 0 0 1 2 2 2
  line L554 (-29.4166, -8.783) -> (-29.4166, -7.8203)
  line L555 (-29.4166, -7.8203) -> (-28.7116, -7.8203)
  line L556 (-28.7116, -7.8203) -> (-28.7116, -10.954)
  line L557 (-29.4166, -10.3316) -> (-29.4166, -9.2206)
  spline S427 degree 2 poles (-29.4166, -9.2206) (-29.4676, -9.1939) (-29.6378, -9.1598) (-29.6986, -9.1598) knots 0 0 0 1 2 2 2
  spline S428 degree 2 poles (-29.6986, -9.1598) (-29.9514, -9.1598) (-30.2067, -9.5148) (-30.2067, -9.8333) knots 0 0 0 1 2 2 2
  spline S429 degree 2 poles (-30.2067, -9.8333) (-30.2067, -10.1688) (-30.0025, -10.4678) (-29.7764, -10.4678) knots 0 0 0 1 2 2 2
  spline S430 degree 2 poles (-29.7764, -10.4678) (-29.684, -10.4678) (-29.4944, -10.3948) (-29.4166, -10.3316) knots 0 0 0 1 2 2 2
  line L558 (-26.6524, -9.3592) -> (-26.7107, -9.3592)
  spline S431 degree 2 poles (-26.7107, -9.3592) (-26.7521, -9.3446) (-26.9052, -9.33) (-26.9976, -9.33) knots 0 0 0 1 2 2 2
  spline S432 degree 2 poles (-26.9976, -9.33) (-27.107, -9.33) (-27.3526, -9.3957) (-27.4668, -9.4394) knots 0 0 0 1 2 2 2
  line L559 (-27.4668, -9.4394) -> (-27.4668, -10.954)
  line L560 (-27.4668, -10.954) -> (-28.1718, -10.954)
  line L561 (-28.1718, -10.954) -> (-28.1718, -8.6906)
  line L562 (-28.1718, -8.6906) -> (-27.4668, -8.6906)
  line L563 (-27.4668, -8.6906) -> (-27.4668, -9.0164)
  spline S433 degree 2 poles (-27.4668, -9.0164) (-27.4182, -8.9726) (-27.248, -8.8365) (-27.1775, -8.7952) knots 0 0 0 1 2 2 2
  spline S434 degree 2 poles (-27.1775, -8.7952) (-27.0997, -8.749) (-26.8955, -8.6833) (-26.8056, -8.6833) knots 0 0 0 1 2 2 2
  spline S435 degree 2 poles (-26.8056, -8.6833) (-26.7715, -8.6833) (-26.6864, -8.6882) (-26.6524, -8.6906) knots 0 0 0 1 2 2 2
  line L564 (-26.6524, -8.6906) -> (-26.6524, -9.3592)
  line L565 (-24.4692, -10.954) -> (-25.1743, -10.954)
  line L566 (-25.1743, -10.954) -> (-25.1743, -8.6906)
  line L567 (-25.1743, -8.6906) -> (-24.4692, -8.6906)
  line L568 (-24.4692, -8.6906) -> (-24.4692, -10.954)
  line L569 (-24.4474, -8.3673) -> (-25.1937, -8.3673)
  line L570 (-25.1937, -8.3673) -> (-25.1937, -7.8179)
  line L571 (-25.1937, -7.8179) -> (-24.4474, -7.8179)
  line L572 (-24.4474, -7.8179) -> (-24.4474, -8.3673)
  line L573 (-21.812, -10.954) -> (-22.5219, -10.954)
  line L574 (-22.5219, -10.954) -> (-22.5219, -9.8333)
  spline S436 degree 2 poles (-22.5219, -9.8333) (-22.5219, -9.6947) (-22.5438, -9.4224) (-22.573, -9.3592) knots 0 0 0 1 2 2 2
  spline S437 degree 2 poles (-22.573, -9.3592) (-22.6094, -9.2814) (-22.7456, -9.2158) (-22.8623, -9.2158) knots 0 0 0 1 2 2 2
  spline S438 degree 2 poles (-22.8623, -9.2158) (-22.9474, -9.2158) (-23.1248, -9.2814) (-23.2245, -9.3519) knots 0 0 0 1 2 2 2
  line L575 (-23.2245, -9.3519) -> (-23.2245, -10.954)
  line L576 (-23.2245, -10.954) -> (-23.9295, -10.954)
  line L577 (-23.9295, -10.954) -> (-23.9295, -8.6906)
  line L578 (-23.9295, -8.6906) -> (-23.2245, -8.6906)
  line L579 (-23.2245, -8.6906) -> (-23.2245, -8.941)
  spline S439 degree 2 poles (-23.2245, -8.941) (-23.0519, -8.7952) (-22.7237, -8.6299) (-22.5244, -8.6299) knots 0 0 0 1 2 2 2
  spline S440 degree 2 poles (-22.5244, -8.6299) (-22.1791, -8.6299) (-21.812, -9.0675) (-21.812, -9.4807) knots 0 0 0 1 2 2 2
  line L580 (-21.812, -9.4807) -> (-21.812, -10.954)
  line L581 (-19.4855, -10.954) -> (-21.462, -10.954)
  line L582 (-21.462, -10.954) -> (-21.462, -10.4897)
  line L583 (-21.462, -10.4897) -> (-20.3825, -9.2206)
  line L584 (-20.3825, -9.2206) -> (-21.4133, -9.2206)
  line L585 (-21.4133, -9.2206) -> (-21.4133, -8.6906)
  line L586 (-21.4133, -8.6906) -> (-19.5073, -8.6906)
  line L587 (-19.5073, -8.6906) -> (-19.5073, -9.1477)
  line L588 (-19.5073, -9.1477) -> (-20.5892, -10.4143)
  line L589 (-20.5892, -10.4143) -> (-19.4855, -10.4143)
  line L590 (-19.4855, -10.4143) -> (-19.4855, -10.954)
  line L591 (-20.0738, -8.3697) -> (-20.7983, -8.3697)
  line L592 (-20.7983, -8.3697) -> (-20.7983, -7.8203)
  line L593 (-20.7983, -7.8203) -> (-20.0738, -7.8203)
  line L594 (-20.0738, -7.8203) -> (-20.0738, -8.3697)
  line L595 (-18.3915, -10.954) -> (-19.1038, -10.954)
  line L596 (-19.1038, -10.954) -> (-19.1038, -10.1615)
  line L597 (-19.1038, -10.1615) -> (-18.3915, -10.1615)
  line L598 (-18.3915, -10.1615) -> (-18.3915, -10.954)
  spline S441 degree 2 poles (-13.906, -9.4564) (-13.906, -9.877) (-14.2731, -10.5383) (-14.5527, -10.7158) knots 0 0 0 1 2 2 2
  spline S442 degree 2 poles (-14.5527, -10.7158) (-14.7861, -10.8665) (-15.3355, -10.954) (-15.6443, -10.954) knots 0 0 0 1 2 2 2
  line L599 (-15.6443, -10.954) -> (-16.5827, -10.954)
  line L600 (-16.5827, -10.954) -> (-16.5827, -7.954)
  line L601 (-16.5827, -7.954) -> (-15.654, -7.954)
  spline S443 degree 2 poles (-15.654, -7.954) (-15.338, -7.954) (-14.7861, -8.0342) (-14.543, -8.1898) knots 0 0 0 1 2 2 2
  spline S444 degree 2 poles (-14.543, -8.1898) (-14.2488, -8.3795) (-13.906, -9.0213) (-13.906, -9.4564) knots 0 0 0 1 2 2 2
  spline S445 degree 2 poles (-14.6791, -9.4516) (-14.6791, -9.155) (-14.8833, -8.732) (-15.0924, -8.6128) knots 0 0 0 1 2 2 2
  spline S446 degree 2 poles (-15.0924, -8.6128) (-15.2456, -8.5302) (-15.5811, -8.5132) (-15.8145, -8.5132) knots 0 0 0 1 2 2 2
  line L602 (-15.8145, -8.5132) -> (-15.8291, -8.5132)
  line L603 (-15.8291, -8.5132) -> (-15.8291, -10.3924)
  line L604 (-15.8291, -10.3924) -> (-15.8145, -10.3924)
  spline S447 degree 2 poles (-15.8145, -10.3924) (-15.5616, -10.3924) (-15.214, -10.3754) (-15.056, -10.2757) knots 0 0 0 1 2 2 2
  spline S448 degree 2 poles (-15.056, -10.2757) (-14.8712, -10.159) (-14.6791, -9.7482) (-14.6791, -9.4516) knots 0 0 0 1 2 2 2
  spline S449 degree 2 poles (-12.2529, -10.7133) (-12.3258, -10.7741) (-12.4401, -10.8713) (-12.5373, -10.92) knots 0 0 0 1 2 2 2
  spline S450 degree 2 poles (-12.5373, -10.92) (-12.6321, -10.9662) (-12.812, -11.0148) (-12.9725, -11.0148) knots 0 0 0 1 2 2 2
  spline S451 degree 2 poles (-12.9725, -11.0148) (-13.2739, -11.0148) (-13.6702, -10.6112) (-13.6702, -10.3049) knots 0 0 0 1 2 2 2
  spline S452 degree 2 poles (-13.6702, -10.3049) (-13.6702, -10.0545) (-13.4684, -9.7433) (-13.2788, -9.6534) knots 0 0 0 1 2 2 2
  spline S453 degree 2 poles (-13.2788, -9.6534) (-13.0868, -9.561) (-12.5543, -9.488) (-12.248, -9.4686) knots 0 0 0 1 2 2 2
  line L605 (-12.248, -9.4686) -> (-12.248, -9.4564)
  spline S454 degree 2 poles (-12.248, -9.4564) (-12.248, -9.2692) (-12.5252, -9.1258) (-12.8023, -9.1258) knots 0 0 0 1 2 2 2
  spline S455 degree 2 poles (-12.8023, -9.1258) (-12.9263, -9.1258) (-13.2618, -9.2158) (-13.4198, -9.2863) knots 0 0 0 1 2 2 2
  line L606 (-13.4198, -9.2863) -> (-13.4806, -9.2863)
  line L607 (-13.4806, -9.2863) -> (-13.4806, -8.7393)
  spline S456 degree 2 poles (-13.4806, -8.7393) (-13.3761, -8.7101) (-12.9093, -8.6274) (-12.671, -8.6274) knots 0 0 0 1 2 2 2
  spline S457 degree 2 poles (-12.671, -8.6274) (-12.0876, -8.6274) (-11.5527, -9.0164) (-11.5527, -9.4151) knots 0 0 0 1 2 2 2
  line L608 (-11.5527, -9.4151) -> (-11.5527, -10.954)
  line L609 (-11.5527, -10.954) -> (-12.2529, -10.954)
  line L610 (-12.2529, -10.954) -> (-12.2529, -10.7133)
  line L611 (-12.2529, -10.3632) -> (-12.2529, -9.894)
  spline S458 degree 2 poles (-12.2529, -9.894) (-12.4328, -9.9111) (-12.654, -9.9378) (-12.761, -9.9767) knots 0 0 0 1 2 2 2
  spline S459 degree 2 poles (-12.761, -9.9767) (-12.8558, -10.0083) (-12.9579, -10.1396) (-12.9579, -10.2466) knots 0 0 0 1 2 2 2
  spline S460 degree 2 poles (-12.9579, -10.2466) (-12.9579, -10.4046) (-12.7853, -10.5237) (-12.6175, -10.5237) knots 0 0 0 1 2 2 2
  spline S461 degree 2 poles (-12.6175, -10.5237) (-12.5252, -10.5237) (-12.3307, -10.4386) (-12.2529, -10.3632) knots 0 0 0 1 2 2 2
  line L612 (-9.5106, -9.3592) -> (-9.5689, -9.3592)
  spline S462 degree 2 poles (-9.5689, -9.3592) (-9.6103, -9.3446) (-9.7634, -9.33) (-9.8558, -9.33) knots 0 0 0 1 2 2 2
  spline S463 degree 2 poles (-9.8558, -9.33) (-9.9652, -9.33) (-10.2107, -9.3957) (-10.325, -9.4394) knots 0 0 0 1 2 2 2
  line L613 (-10.325, -9.4394) -> (-10.325, -10.954)
  line L614 (-10.325, -10.954) -> (-11.03, -10.954)
  line L615 (-11.03, -10.954) -> (-11.03, -8.6906)
  line L616 (-11.03, -8.6906) -> (-10.325, -8.6906)
  line L617 (-10.325, -8.6906) -> (-10.325, -9.0164)
  spline S464 degree 2 poles (-10.325, -9.0164) (-10.2764, -8.9726) (-10.1062, -8.8365) (-10.0357, -8.7952) knots 0 0 0 1 2 2 2
  spline S465 degree 2 poles (-10.0357, -8.7952) (-9.9579, -8.749) (-9.7537, -8.6833) (-9.6637, -8.6833) knots 0 0 0 1 2 2 2
  spline S466 degree 2 poles (-9.6637, -8.6833) (-9.6297, -8.6833) (-9.5446, -8.6882) (-9.5106, -8.6906) knots 0 0 0 1 2 2 2
  line L618 (-9.5106, -8.6906) -> (-9.5106, -9.3592)
  line L619 (-8.5357, -10.954) -> (-9.2407, -10.954)
  line L620 (-9.2407, -10.954) -> (-9.2407, -8.6906)
  line L621 (-9.2407, -8.6906) -> (-8.5357, -8.6906)
  line L622 (-8.5357, -8.6906) -> (-8.5357, -10.954)
  line L623 (-8.5138, -8.3673) -> (-9.2602, -8.3673)
  line L624 (-9.2602, -8.3673) -> (-9.2602, -7.8179)
  line L625 (-9.2602, -7.8179) -> (-8.5138, -7.8179)
  line L626 (-8.5138, -7.8179) -> (-8.5138, -8.3673)
  line L627 (-5.8955, -10.954) -> (-6.6005, -10.954)
  line L628 (-6.6005, -10.954) -> (-6.6005, -10.7036)
  spline S467 degree 2 poles (-6.6005, -10.7036) (-6.7829, -10.8568) (-7.0892, -11.0172) (-7.3007, -11.0172) knots 0 0 0 1 2 2 2
  spline S468 degree 2 poles (-7.3007, -11.0172) (-7.6362, -11.0172) (-8.013, -10.5918) (-8.013, -10.1639) knots 0 0 0 1 2 2 2
  line L629 (-8.013, -10.1639) -> (-8.013, -8.6906)
  line L630 (-8.013, -8.6906) -> (-7.3031, -8.6906)
  line L631 (-7.3031, -8.6906) -> (-7.3031, -9.8138)
  spline S469 degree 2 poles (-7.3031, -9.8138) (-7.3031, -9.9889) (-7.2861, -10.2125) (-7.2521, -10.2879) knots 0 0 0 1 2 2 2
  spline S470 degree 2 poles (-7.2521, -10.2879) (-7.218, -10.3584) (-7.0843, -10.4313) (-6.9628, -10.4313) knots 0 0 0 1 2 2 2
  spline S471 degree 2 poles (-6.9628, -10.4313) (-6.8898, -10.4313) (-6.6856, -10.3584) (-6.6005, -10.2952) knots 0 0 0 1 2 2 2
  line L632 (-6.6005, -10.2952) -> (-6.6005, -8.6906)
  line L633 (-6.6005, -8.6906) -> (-5.8955, -8.6906)
  line L634 (-5.8955, -8.6906) -> (-5.8955, -10.954)
  spline S472 degree 2 poles (-4.6678, -11.0148) (-4.9158, -11.0148) (-5.3607, -10.9054) (-5.5065, -10.8325) knots 0 0 0 1 2 2 2
  line L635 (-5.5065, -10.8325) -> (-5.5065, -10.2368)
  line L636 (-5.5065, -10.2368) -> (-5.4482, -10.2368)
  spline S473 degree 2 poles (-5.4482, -10.2368) (-5.3971, -10.2757) (-5.2683, -10.3681) (-5.154, -10.4192) knots 0 0 0 1 2 2 2
  spline S474 degree 2 poles (-5.154, -10.4192) (-5.0543, -10.4654) (-4.8088, -10.531) (-4.6629, -10.531) knots 0 0 0 1 2 2 2
  spline S475 degree 2 poles (-4.6629, -10.531) (-4.5146, -10.531) (-4.2861, -10.4386) (-4.2861, -10.3389) knots 0 0 0 1 2 2 2
  spline S476 degree 2 poles (-4.2861, -10.3389) (-4.2861, -10.2611) (-4.3906, -10.1785) (-4.5414, -10.1444) knots 0 0 0 1 2 2 2
  spline S477 degree 2 poles (-4.5414, -10.1444) (-4.6216, -10.1226) (-4.8671, -10.0764) (-4.962, -10.0472) knots 0 0 0 1 2 2 2
  spline S478 degree 2 poles (-4.962, -10.0472) (-5.2294, -9.9645) (-5.4968, -9.6412) (-5.4968, -9.3762) knots 0 0 0 1 2 2 2
  spline S479 degree 2 poles (-5.4968, -9.3762) (-5.4968, -9.2255) (-5.3582, -8.9581) (-5.2221, -8.8535) knots 0 0 0 1 2 2 2
  spline S480 degree 2 poles (-5.2221, -8.8535) (-5.0884, -8.7514) (-4.6921, -8.6299) (-4.4417, -8.6299) knots 0 0 0 1 2 2 2
  spline S481 degree 2 poles (-4.4417, -8.6299) (-4.2034, -8.6299) (-3.8047, -8.7247) (-3.6686, -8.7903) knots 0 0 0 1 2 2 2
  line L637 (-3.6686, -8.7903) -> (-3.6686, -9.3641)
  line L638 (-3.6686, -9.3641) -> (-3.7245, -9.3641)
  spline S482 degree 2 poles (-3.7245, -9.3641) (-3.761, -9.3349) (-3.919, -9.2401) (-3.9919, -9.206) knots 0 0 0 1 2 2 2
  spline S483 degree 2 poles (-3.9919, -9.206) (-4.0819, -9.1671) (-4.3007, -9.1136) (-4.415, -9.1136) knots 0 0 0 1 2 2 2
  spline S484 degree 2 poles (-4.415, -9.1136) (-4.5681, -9.1136) (-4.7796, -9.2182) (-4.7796, -9.3033) knots 0 0 0 1 2 2 2
  spline S485 degree 2 poles (-4.7796, -9.3033) (-4.7796, -9.3811) (-4.6751, -9.4686) (-4.5, -9.5124) knots 0 0 0 1 2 2 2
  spline S486 degree 2 poles (-4.5, -9.5124) (-4.4101, -9.5342) (-4.1743, -9.5756) (-4.0649, -9.612) knots 0 0 0 1 2 2 2
  spline S487 degree 2 poles (-4.0649, -9.612) (-3.8218, -9.6898) (-3.5689, -9.9937) (-3.5689, -10.2466) knots 0 0 0 1 2 2 2
  spline S488 degree 2 poles (-3.5689, -10.2466) (-3.5689, -10.4046) (-3.7172, -10.6939) (-3.8558, -10.7911) knots 0 0 0 1 2 2 2
  spline S489 degree 2 poles (-3.8558, -10.7911) (-3.9992, -10.8981) (-4.3931, -11.0148) (-4.6678, -11.0148) knots 0 0 0 1 2 2 2
  line L639 (-1.4295, -10.954) -> (-3.406, -10.954)
  line L640 (-3.406, -10.954) -> (-3.406, -10.4897)
  line L641 (-3.406, -10.4897) -> (-2.3266, -9.2206)
  line L642 (-2.3266, -9.2206) -> (-3.3574, -9.2206)
  line L643 (-3.3574, -9.2206) -> (-3.3574, -8.6906)
  line L644 (-3.3574, -8.6906) -> (-1.4514, -8.6906)
  line L645 (-1.4514, -8.6906) -> (-1.4514, -9.1477)
  line L646 (-1.4514, -9.1477) -> (-2.5333, -10.4143)
  line L647 (-2.5333, -10.4143) -> (-1.4295, -10.4143)
  line L648 (-1.4295, -10.4143) -> (-1.4295, -10.954)
  spline S490 degree 2 poles (0.1823, -10.7133) (0.1094, -10.7741) (-0.0049, -10.8713) (-0.1021, -10.92) knots 0 0 0 1 2 2 2
  spline S491 degree 2 poles (-0.1021, -10.92) (-0.197, -10.9662) (-0.3769, -11.0148) (-0.5373, -11.0148) knots 0 0 0 1 2 2 2
  spline S492 degree 2 poles (-0.5373, -11.0148) (-0.8388, -11.0148) (-1.2351, -10.6112) (-1.2351, -10.3049) knots 0 0 0 1 2 2 2
  spline S493 degree 2 poles (-1.2351, -10.3049) (-1.2351, -10.0545) (-1.0333, -9.7433) (-0.8436, -9.6534) knots 0 0 0 1 2 2 2
  spline S494 degree 2 poles (-0.8436, -9.6534) (-0.6516, -9.561) (-0.1192, -9.488) (0.1872, -9.4686) knots 0 0 0 1 2 2 2
  line L649 (0.1872, -9.4686) -> (0.1872, -9.4564)
  spline S495 degree 2 poles (0.1872, -9.4564) (0.1872, -9.2692) (-0.09, -9.1258) (-0.3671, -9.1258) knots 0 0 0 1 2 2 2
  spline S496 degree 2 poles (-0.3671, -9.1258) (-0.4911, -9.1258) (-0.8266, -9.2158) (-0.9846, -9.2863) knots 0 0 0 1 2 2 2
  line L650 (-0.9846, -9.2863) -> (-1.0454, -9.2863)
  line L651 (-1.0454, -9.2863) -> (-1.0454, -8.7393)
  spline S497 degree 2 poles (-1.0454, -8.7393) (-0.9409, -8.7101) (-0.4741, -8.6274) (-0.2359, -8.6274) knots 0 0 0 1 2 2 2
  spline S498 degree 2 poles (-0.2359, -8.6274) (0.3476, -8.6274) (0.8825, -9.0164) (0.8825, -9.4151) knots 0 0 0 1 2 2 2
  line L652 (0.8825, -9.4151) -> (0.8825, -10.954)
  line L653 (0.8825, -10.954) -> (0.1823, -10.954)
  line L654 (0.1823, -10.954) -> (0.1823, -10.7133)
  line L655 (0.1823, -10.3632) -> (0.1823, -9.894)
  spline S499 degree 2 poles (0.1823, -9.894) (0.0024, -9.9111) (-0.2188, -9.9378) (-0.3258, -9.9767) knots 0 0 0 1 2 2 2
  spline S500 degree 2 poles (-0.3258, -9.9767) (-0.4206, -10.0083) (-0.5227, -10.1396) (-0.5227, -10.2466) knots 0 0 0 1 2 2 2
  spline S501 degree 2 poles (-0.5227, -10.2466) (-0.5227, -10.4046) (-0.3501, -10.5237) (-0.1824, -10.5237) knots 0 0 0 1 2 2 2
  spline S502 degree 2 poles (-0.1824, -10.5237) (-0.09, -10.5237) (0.1045, -10.4386) (0.1823, -10.3632) knots 0 0 0 1 2 2 2
  line L656 (5.7179, -10.954) -> (4.9692, -10.954)
  line L657 (4.9692, -10.954) -> (4.9692, -8.9654)
  line L658 (4.9692, -8.9654) -> (4.4246, -10.249)
  line L659 (4.4246, -10.249) -> (3.9092, -10.249)
  line L660 (3.9092, -10.249) -> (3.3646, -8.9654)
  line L661 (3.3646, -8.9654) -> (3.3646, -10.954)
  line L662 (3.3646, -10.954) -> (2.6547, -10.954)
  line L663 (2.6547, -10.954) -> (2.6547, -7.954)
  line L664 (2.6547, -7.954) -> (3.5226, -7.954)
  line L665 (3.5226, -7.954) -> (4.1888, -9.4346)
  line L666 (4.1888, -9.4346) -> (4.85, -7.954)
  line L667 (4.85, -7.954) -> (5.7179, -7.954)
  line L668 (5.7179, -7.954) -> (5.7179, -10.954)
  spline S503 degree 2 poles (8.47, -9.8235) (8.47, -10.3827) (7.8598, -11.0245) (7.303, -11.0245) knots 0 0 0 1 2 2 2
  spline S504 degree 2 poles (7.303, -11.0245) (6.7487, -11.0245) (6.1337, -10.3827) (6.1337, -9.8235) knots 0 0 0 1 2 2 2
  spline S505 degree 2 poles (6.1337, -9.8235) (6.1337, -9.2595) (6.7487, -8.6201) (7.303, -8.6201) knots 0 0 0 1 2 2 2
  spline S506 degree 2 poles (7.303, -8.6201) (7.8573, -8.6201) (8.47, -9.2619) (8.47, -9.8235) knots 0 0 0 1 2 2 2
  spline S507 degree 2 poles (7.7479, -9.8284) (7.7479, -9.6266) (7.6823, -9.3568) (7.6239, -9.2765) knots 0 0 0 1 2 2 2
  spline S508 degree 2 poles (7.6239, -9.2765) (7.5607, -9.1914) (7.4027, -9.1258) (7.303, -9.1258) knots 0 0 0 1 2 2 2
  spline S509 degree 2 poles (7.303, -9.1258) (7.2058, -9.1258) (7.0526, -9.1842) (6.9894, -9.2668) knots 0 0 0 1 2 2 2
  spline S510 degree 2 poles (6.9894, -9.2668) (6.9286, -9.3446) (6.8557, -9.6193) (6.8557, -9.8284) knots 0 0 0 1 2 2 2
  spline S511 degree 2 poles (6.8557, -9.8284) (6.8557, -10.035) (6.9238, -10.2903) (6.9797, -10.3681) knots 0 0 0 1 2 2 2
  spline S512 degree 2 poles (6.9797, -10.3681) (7.0356, -10.4459) (7.2058, -10.5188) (7.3079, -10.5188) knots 0 0 0 1 2 2 2
  spline S513 degree 2 poles (7.3079, -10.5188) (7.393, -10.5188) (7.568, -10.4459) (7.6215, -10.373) knots 0 0 0 1 2 2 2
  spline S514 degree 2 poles (7.6215, -10.373) (7.6823, -10.2879) (7.7479, -10.0423) (7.7479, -9.8284) knots 0 0 0 1 2 2 2
  spline S515 degree 2 poles (9.5324, -11.0148) (9.2844, -11.0148) (8.8395, -10.9054) (8.6936, -10.8325) knots 0 0 0 1 2 2 2
  line L669 (8.6936, -10.8325) -> (8.6936, -10.2368)
  line L670 (8.6936, -10.2368) -> (8.752, -10.2368)